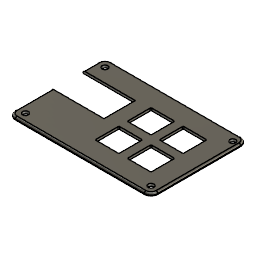
hackpad top plate (Autodesk Fusion 360 design; units mm, degrees)
Autodesk Fusion 360 part; units mm, degrees
sketch "plate-2025-12-03T19_15_09.193Z" plane through (0, 0, 0) normal (0, 0, 1) x (1, 0, 0)
  line L0 (3.025, -21.575) -> (16.025, -21.575)
  line L1 (3.025, -35.575) -> (16.025, -35.575)
  line L2 (2.525, -22.075) -> (2.525, -35.075)
  line L3 (16.525, -22.075) -> (16.525, -35.075)
  arc A0 (3.025, -21.575) -> (2.525, -22.075) centre (3.025, -22.075) ccw
  arc A1 (16.525, -22.075) -> (16.025, -21.575) centre (16.025, -22.075) ccw
  arc A2 (2.525, -35.075) -> (3.025, -35.575) centre (3.025, -35.075) ccw
  arc A3 (16.025, -35.575) -> (16.525, -35.075) centre (16.025, -35.075) ccw
  line L4 (22.075, -21.575) -> (35.075, -21.575)
  line L5 (22.075, -35.575) -> (35.075, -35.575)
  line L6 (21.575, -22.075) -> (21.575, -35.075)
  line L7 (35.575, -22.075) -> (35.575, -35.075)
  arc A4 (22.075, -21.575) -> (21.575, -22.075) centre (22.075, -22.075) ccw
  arc A5 (35.575, -22.075) -> (35.075, -21.575) centre (35.075, -22.075) ccw
  arc A6 (21.575, -35.075) -> (22.075, -35.575) centre (22.075, -35.075) ccw
  arc A7 (35.075, -35.575) -> (35.575, -35.075) centre (35.075, -35.075) ccw
  line L8 (3.025, -40.625) -> (16.025, -40.625)
  line L9 (3.025, -54.625) -> (16.025, -54.625)
  line L10 (2.525, -41.125) -> (2.525, -54.125)
  line L11 (16.525, -41.125) -> (16.525, -54.125)
  arc A8 (3.025, -40.625) -> (2.525, -41.125) centre (3.025, -41.125) ccw
  arc A9 (16.525, -41.125) -> (16.025, -40.625) centre (16.025, -41.125) ccw
  arc A10 (2.525, -54.125) -> (3.025, -54.625) centre (3.025, -54.125) ccw
  arc A11 (16.025, -54.625) -> (16.525, -54.125) centre (16.025, -54.125) ccw
  line L12 (22.075, -40.625) -> (35.075, -40.625)
  line L13 (22.075, -54.625) -> (35.075, -54.625)
  line L14 (21.575, -41.125) -> (21.575, -54.125)
  line L15 (35.575, -41.125) -> (35.575, -54.125)
  arc A12 (22.075, -40.625) -> (21.575, -41.125) centre (22.075, -41.125) ccw
  arc A13 (35.575, -41.125) -> (35.075, -40.625) centre (35.075, -41.125) ccw
  arc A14 (21.575, -54.125) -> (22.075, -54.625) centre (22.075, -54.125) ccw
  arc A15 (35.075, -54.625) -> (35.575, -54.125) centre (35.075, -54.125) ccw
  line L16 (-36.785, -9.535) -> (47.615, -9.535)
  line L17 (47.615, -9.535) -> (47.615, -66.665)
  line L18 (47.615, -66.665) -> (-36.785, -66.665)
  line L19 (-36.785, -66.665) -> (-36.785, -9.535)
  line L20 (-36.785, -22.615) -> (-5.785, -22.615)
  line L21 (-5.785, -22.615) -> (-5.785, -41.115)
  line L22 (-5.785, -41.115) -> (-36.785, -41.115)
  line L23 (-36.785, -41.115) -> (-36.785, -22.615)
  circle A16 centre (-31.785, -14.535) radius 1.7
  circle A17 centre (-31.785, -61.665) radius 1.7
  circle A18 centre (42.615, -61.665) radius 1.7
  circle A19 centre (44, -14.535) radius 1.7
  dimension "d1" = 12.04
  dimension "d3" = 12.04
  dimension "d4" = 12.04
  dimension "d5" = 84.4
  dimension "d6" = 18.5
  dimension "d7" = 31
  dimension "d8" = 25.55
  dimension "d9" = 3.4
  dimension "d10" = 3.4
  dimension "d11" = 3.4
  dimension "d12" = 3.4
  dimension "d13" = 5
  dimension "d14" = 5
  dimension "d15" = 5
  dimension "d16" = 5
  dimension "d17" = 5
  dimension "d18" = 5
  dimension "d19" = 5
  dimension "d20" = 3.615
  constraint horizontal L16
  constraint vertical L17
  constraint horizontal L18
  constraint vertical L19
  constraint horizontal L20
  constraint vertical L21
  constraint horizontal L22
  constraint vertical L23
  constraint coincident L19 L20.start
  measures "d1" distance of L9 L18
  measures "d3" distance of L15 L17
  measures "d4" distance of L4 L16
  measures "d5" distance of L17 L19
  measures "d6" distance of L20.start L22.end
  measures "d7" distance of L21 L23
  measures "d8" distance of L18 L22
  measures "d9" diameter of A16
  measures "d10" diameter of A17
  measures "d11" diameter of A18
  measures "d12" diameter of A19
  measures "d13" distance of L16 A16.centre
  measures "d14" distance of L19 A16.centre
  measures "d15" distance of L19 A17.centre
  measures "d16" distance of L18 A17.centre
  measures "d17" distance of L18 A18.centre
  measures "d18" distance of L17 A18.centre
  measures "d19" distance of L16 A19.centre
  measures "d20" distance of L17 A19.centre
extrude "Extrude1" add sketch "plate-2025-12-03T19_15_09.193Z" along normal blind 1.5 contours L16 L17 L18 L19 L20 L21 L22
fillet "Fillet1" radius 4 4 edges at (47.615, -66.665, 0.75) (47.615, -9.535, 0.75) (-36.785, -9.535, 0.75) (-36.785, -66.665, 0.75)
fillet "Fillet2" radius 1 9 edges at (-36.785, -51.89, 1.5) (-35.6134, -65.4934, 1.5) (5.415, -66.665, 1.5) (46.4434, -65.4934, 1.5) (47.615, -38.1, 1.5) (46.4434, -10.7066, 1.5) (5.415, -9.535, 1.5) (-35.6134, -10.7066, 1.5) (-36.785, -18.075, 1.5)
sketch "Sketch2" plane through (0, 0, 0) normal (0, 0, -1) x (1, 0, 0)
  circle A0 centre (42.615, 61.665) radius 1.7
  arc A1 (21.575, 41.125) -> (22.075, 40.625) centre (22.075, 41.125) ccw
  line L0 (21.575, 41.125) -> (21.575, 54.125)
  arc A2 (22.075, 54.625) -> (21.575, 54.125) centre (22.075, 54.125) ccw
  line L1 (22.075, 54.625) -> (35.075, 54.625)
  arc A3 (35.575, 54.125) -> (35.075, 54.625) centre (35.075, 54.125) ccw
  line L2 (35.575, 54.125) -> (35.575, 41.125)
  arc A4 (35.075, 40.625) -> (35.575, 41.125) centre (35.075, 41.125) ccw
  line L3 (35.075, 40.625) -> (22.075, 40.625)
  circle A5 centre (-31.785, 61.665) radius 1.7
  arc A6 (21.575, 22.075) -> (22.075, 21.575) centre (22.075, 22.075) ccw
  line L4 (21.575, 22.075) -> (21.575, 35.075)
  arc A7 (22.075, 35.575) -> (21.575, 35.075) centre (22.075, 35.075) ccw
  line L5 (22.075, 35.575) -> (35.075, 35.575)
  arc A8 (35.575, 35.075) -> (35.075, 35.575) centre (35.075, 35.075) ccw
  line L6 (35.575, 35.075) -> (35.575, 22.075)
  arc A9 (35.075, 21.575) -> (35.575, 22.075) centre (35.075, 22.075) ccw
  line L7 (35.075, 21.575) -> (22.075, 21.575)
  circle A10 centre (-31.785, 14.535) radius 1.7
  circle A11 centre (44, 14.535) radius 1.7
  arc A12 (2.525, 22.075) -> (3.025, 21.575) centre (3.025, 22.075) ccw
  line L8 (2.525, 22.075) -> (2.525, 35.075)
  arc A13 (3.025, 35.575) -> (2.525, 35.075) centre (3.025, 35.075) ccw
  line L9 (3.025, 35.575) -> (16.025, 35.575)
  arc A14 (16.525, 35.075) -> (16.025, 35.575) centre (16.025, 35.075) ccw
  line L10 (16.525, 35.075) -> (16.525, 22.075)
  arc A15 (16.025, 21.575) -> (16.525, 22.075) centre (16.025, 22.075) ccw
  line L11 (16.025, 21.575) -> (3.025, 21.575)
  arc A16 (2.525, 41.125) -> (3.025, 40.625) centre (3.025, 41.125) ccw
  line L12 (2.525, 41.125) -> (2.525, 54.125)
  arc A17 (3.025, 54.625) -> (2.525, 54.125) centre (3.025, 54.125) ccw
  line L13 (3.025, 54.625) -> (16.025, 54.625)
  arc A18 (16.525, 54.125) -> (16.025, 54.625) centre (16.025, 54.125) ccw
  line L14 (16.525, 54.125) -> (16.525, 41.125)
  arc A19 (16.025, 40.625) -> (16.525, 41.125) centre (16.025, 41.125) ccw
  line L15 (16.025, 40.625) -> (3.025, 40.625)
  arc A20 (-32.785, 66.665) -> (-36.785, 62.665) centre (-32.785, 62.665) ccw
  line L16 (-36.785, 62.665) -> (-36.785, 41.115)
  line L17 (-36.785, 41.115) -> (-5.785, 41.115)
  line L18 (-5.785, 41.115) -> (-5.785, 22.615)
  line L19 (-5.785, 22.615) -> (-36.785, 22.615)
  line L20 (-36.785, 22.615) -> (-36.785, 13.535)
  arc A21 (-36.785, 13.535) -> (-32.785, 9.535) centre (-32.785, 13.535) ccw
  line L21 (-32.785, 9.535) -> (43.615, 9.535)
  arc A22 (43.615, 9.535) -> (47.615, 13.535) centre (43.615, 13.535) ccw
  line L22 (47.615, 13.535) -> (47.615, 62.665)
  arc A23 (47.615, 62.665) -> (43.615, 66.665) centre (43.615, 62.665) ccw
  line L23 (43.615, 66.665) -> (-32.785, 66.665)
  line L24 (-30.063, 52.1514) -> (-16, 52) construction
  line L25 (-16, 52) -> (-15.937, 57.8486) construction
  line L26 (-15.937, 57.8486) -> (-30, 58) construction
  line L27 (-30, 58) -> (-30.063, 52.1514) construction
  dimension "d27" = 3
  text T0 "Hackpad by nilslm" font "Arial" height 3 align left top in box 14.0638 x 5.8489 at (-30.063, 52.1514) x (0.999942, -0.010768) y (0.010768, 0.999942) spacing 1
extrude "Extrude2" cut sketch "Sketch2" against normal blind 0.2 text T0
equation "d1 = 2.540 mm + 9.5 mm"
equation "d3 = 2.540 mm + 9.5 mm"
equation "d4 = 2.540 mm + 9.5 mm"
equation "d8 = 19.80 mm + 5.75 mm"
equation "d28 = 'Hackpad by nilslm'"
